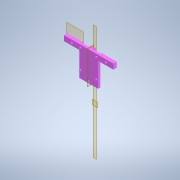
# Autodesk Inventor part: STM_Rear
Saved by Autodesk Inventor 2020 (Build 240168000, 168)
## iProperties
Created: 2022-10-27
Part Number: STM_Rear
Material: 일반
Document SubType Name: Modeling
Designer: ASUS
Density: 1 g/cm^3
Appearance: 기본값
Author: ASUS
Autodesk Inventor part; units mm, degrees
ref_plane "YZ Plane" through (0, 0, 0) normal (1, 0, 0) x (0, 1, 0)
ref_plane "작업 평면1" through (0, 0, 0) normal (0, 0, 1) x (1, 0, 0)
sketch "스케치1" plane through (0, 0, 0) normal (0, 0, 1) x (1, 0, 0)
  line L0 (18, -188.5) -> (18, 261.5) projected
  line L1 (-62, 170.2) -> (-62, 0) projected
  line L2 (-62, -188.5) -> (-62, 261.5) projected
  line L3 (163.5, 192.5) -> (-207.5, 192.5) projected
  line L4 (-32, 167.5) -> (-12, 167.5) projected
  line L5 (-12, 167.5) -> (-12, 192.5) projected
  line L6 (-32, 192.5) -> (-32, 167.5) projected
  line L7 (-12, -188.5) -> (-12, 261.5) projected
  line L8 (-32, -188.5) -> (-32, 261.5) projected
  line L9 (-32, 62) -> (-12, 62) projected
  line L10 (-62, 62.2) -> (18, 62.2)
  line L11 (18, 62.2) -> (18, 192.5)
  line L12 (18, 192.5) -> (-62, 192.5)
  line L13 (-62, 192.5) -> (-62, 62.2)
  point P0 (0, 0)
  point P1 (-62, 192.5)
  dimension "d0" = 0.2
  constraints: 8 end point, 3 point on line, 2 parallel, 1 horizontal, 1 perpendicular
  measures "d0" distance between parallel lines of L9 L10
extrude "돌출1" add sketch "스케치1" along normal blind 10 contours L10 L7 L5 L3 L0 | L10 L8 L4 L7 | L5 L4 L6 L3 | L10 L1 L2 L3 L6 L8
ref_plane "작업 평면2" through (-62, 228.54, -4.7) normal (0, 0, 1) x (0, -1, 0)
sketch "스케치2" plane through (-62, 228.54, -4.7) normal (0, 0, 1) x (0, -1, 0)
  circle A0 centre (15.0001, -54) radius 2.25 projected
  circle A1 centre (15.0001, -13) radius 2.25 projected
  line L0 (68.34, 0) -> (0, 0) projected
  line L1 (68.34, 0) -> (68.34, -67) projected
  line L2 (68.34, -67) -> (0, -67) projected
  line L3 (0, 0) -> (0, -67) projected
  circle A2 centre (15.0001, -54) radius 4 projected
  circle A3 centre (15.0001, -13) radius 4 projected
  line L4 (0, 0) -> (58.34, 0) projected
  line L5 (0, 0) -> (0, -67) projected
  line L6 (0, -67) -> (58.34, -67) projected
  line L7 (58.34, 0) -> (58.34, -67) projected
  circle A4 centre (15.0001, 134) radius 4 projected
  circle A5 centre (15.0001, 93) radius 4 projected
  line L8 (0, 80) -> (58.34, 80) projected
  line L9 (58.34, 80) -> (58.34, 147) projected
  line L10 (0, 147) -> (58.34, 147) projected
  line L11 (0, 80) -> (0, 147) projected
  line L12 (36.04, 225.5) -> (36.04, -145.5) projected
  point P0 (228.54, 62)
  point P1 (36.04, 147)
  point P2 (36.04, 80)
  point P3 (36.04, 0)
  point P4 (36.04, -67)
extrude "돌출2" add sketch "스케치2" along normal up to surface (14.7 mm away) contours L7 L2 L12 L0 | L12 L10 L9 L8
sketch "스케치3" plane through (0, 0, 10) normal (0, 0, 1) x (1, 0, 0)
  line L0 (18, 62.2) -> (18, 170.2) projected
  line L1 (85, 170.2) -> (18, 170.2) projected
  line L2 (85, 192.5) -> (85, 170.2) projected
  line L3 (-129, 192.5) -> (85, 192.5) projected
  line L4 (-129, 170.2) -> (-129, 192.5) projected
  line L5 (-62, 170.2) -> (-129, 170.2) projected
  line L6 (-62, 170.2) -> (-62, 62.2) projected
  line L7 (-62, 62.2) -> (18, 62.2) projected
  circle A0 centre (-95.5, 181.35) radius 4
  line L8 (-97.8094, 177.35) -> (-100.1188, 181.35)
  line L9 (-100.1188, 181.35) -> (-97.8094, 185.35)
  line L10 (-97.8094, 185.35) -> (-93.1906, 185.35)
  line L11 (-93.1906, 185.35) -> (-90.8812, 181.35)
  line L12 (-90.8812, 181.35) -> (-93.1906, 177.35)
  line L13 (-93.1906, 177.35) -> (-97.8094, 177.35)
  circle A1 centre (-22, 70.2) radius 4
  line L14 (-24.3094, 66.2) -> (-26.6188, 70.2)
  line L15 (-26.6188, 70.2) -> (-24.3094, 74.2)
  line L16 (-24.3094, 74.2) -> (-19.6906, 74.2)
  line L17 (-19.6906, 74.2) -> (-17.3812, 70.2)
  line L18 (-17.3812, 70.2) -> (-19.6906, 66.2)
  line L19 (-19.6906, 66.2) -> (-24.3094, 66.2)
  line L20 (18, 62.2) -> (18, 170.2) projected
  line L21 (18, 62.2) -> (-62, 62.2)
  line L22 (-62, 170.2) -> (-129, 170.2) projected
  line L23 (-129, 170.2) -> (-129, 192.5) projected
  line L24 (-62, 170.2) -> (-129, 170.2)
  line L25 (-129, 170.2) -> (-129, 192.5)
  point P0 (0, 0)
  point P1 (-95.5, 177.35)
  point P2 (-22, 66.2)
  point P3 (-129, 181.35)
  point P4 (-129, 181.35)
  point P5 (-22, 62.2)
  point P6 (-95.5, 170.2)
  dimension "d5" = 8
  dimension "d6" = 8
  dimension "d7" = 8
  constraints: 30 end point, 6 midpoint, 4 vertical alignment, 2 coincident, 2 horizontal alignment, 2 perpendicular, 1 collinear, 30 other
  measures "d7" distance from line of L7 point (-22, 70.2)
sketch "스케치4" plane through (0, 0, 0) normal (0, 0, -1) x (-1, 0, 0)
  line L0 (32, 62) -> (12, 62) projected
  line L1 (12, 62) -> (12, 198.5399) projected
  line L2 (32, 198.5399) -> (12, 198.5399) projected
  line L3 (32, 62) -> (32, 198.5399) projected
  line L4 (-18, 62.2) -> (-18, 170.2) projected
  line L5 (-85, 170.2) -> (-18, 170.2) projected
  line L6 (-85, 192.5) -> (-85, 170.2) projected
  line L7 (129, 192.5) -> (-85, 192.5) projected
  line L8 (129, 170.2) -> (129, 192.5) projected
  line L9 (62, 170.2) -> (129, 170.2) projected
  line L10 (62, 170.2) -> (62, 62.2) projected
  line L11 (62, 62.2) -> (-18, 62.2) projected
  circle A0 centre (22, 70.2) radius 2.25 projected
  point P0 (0, 0)
  point P1 (12, 62.2)
  point P2 (32, 62.2)
  point P3 (32, 192.5)
  point P4 (12, 192.5)
ref_plane "작업 평면3" through (-32, 62, -10) normal (0, 0, 1) x (1, 0, 0)
extrude "돌출4" add sketch "스케치4" along normal up to surface (10 mm away) contours L11 L1 L7 L3 | A0
ref_plane "작업 평면4" through (0, 0, 5.8) normal (0, 0, 1) x (1, 0, 0)
sketch "스케치5" plane through (0, 0, 5.8) normal (0, 0, 1) x (1, 0, 0)
  line L0 (18, 62.2) -> (18, 170.2) projected
  line L1 (85, 170.2) -> (18, 170.2) projected
  line L2 (85, 192.5) -> (85, 170.2) projected
  line L3 (-129, 192.5) -> (85, 192.5) projected
  line L4 (-129, 170.2) -> (-129, 192.5) projected
  line L5 (-62, 170.2) -> (-129, 170.2) projected
  line L6 (-62, 170.2) -> (-62, 62.2) projected
  line L7 (-62, 62.2) -> (18, 62.2) projected
  circle A0 centre (-22, 70.2) radius 4
  line L8 (-24.3094, 74.2) -> (-26.6188, 70.2) projected
  circle A1 centre (-95.5, 181.35) radius 4
  point P0 (0, 0)
  constraints: 2 centre point, 1 tangent
hole "구멍1" at (-95.5, 181.35, 5.8) direction (0, 0, -1) diameter 4.5 end through all clearance for "Socket Head Cap Screw ISO 4762" size "M4" standard "ISO"
sketch "스케치6" plane through (0, 0, 0) normal (0, 0, -1) x (-1, 0, 0)
  circle A0 centre (56.5, 98.5) radius 3
  circle A1 centre (56.5, 182.5) radius 3
  line L0 (32, 192.5) -> (62, 192.5) projected
  line L1 (62, 170.2) -> (62, 62.2) projected
  line L2 (53.0359, 98.5) -> (54.7679, 101.5)
  line L3 (54.7679, 101.5) -> (58.2321, 101.5)
  line L4 (58.2321, 101.5) -> (59.9641, 98.5)
  line L5 (59.9641, 98.5) -> (58.2321, 95.5)
  line L6 (58.2321, 95.5) -> (54.7679, 95.5)
  line L7 (54.7679, 95.5) -> (53.0359, 98.5)
  line L8 (54.7679, 179.5) -> (53.0359, 182.5)
  line L9 (53.0359, 182.5) -> (54.7679, 185.5)
  line L10 (54.7679, 185.5) -> (58.2321, 185.5)
  line L11 (58.2321, 185.5) -> (59.9641, 182.5)
  line L12 (59.9641, 182.5) -> (58.2321, 179.5)
  line L13 (58.2321, 179.5) -> (54.7679, 179.5)
  point P0 (0, 0)
  point P1 (53.9019, 97)
  point P2 (56.5, 179.5)
  point P3 (56.5, 95.5)
  dimension "d20" = 6
  dimension "d19" = 84
  dimension "d21" = 10
  dimension "d22" = 5.5
  constraints: 24 end point, 3 midpoint, 3 vertical alignment, 2 coincident, 1 horizontal, 31 other
  measures "d19" distance of point (56.5, 182.5) point (56.5, 98.5)
  measures "d21" distance from line of L0 point (56.5, 182.5)
  measures "d22" distance from line of L1 point (56.5, 98.5)
extrude "돌출5" cut sketch "스케치6" against normal blind 5.2
extrude "돌출6" cut sketch "스케치3" against normal blind 8 contours A0 | A0 L11 L12 | A0 L10 L11 | L12 L13 A0 | A0 L9 L10 | L13 L8 A0 | A0 L8 L9
sketch "스케치7" plane through (0, 0, 10) normal (0, 0, 1) x (1, 0, 0)
  line L0 (-58.2321, 101.5) -> (-59.9641, 98.5) projected
  line L1 (-59.9641, 98.5) -> (-58.2321, 95.5) projected
  line L2 (-58.2321, 95.5) -> (-54.7679, 95.5) projected
  line L3 (-54.7679, 95.5) -> (-53.0359, 98.5) projected
  line L4 (-53.0359, 98.5) -> (-54.7679, 101.5) projected
  line L5 (-54.7679, 101.5) -> (-58.2321, 101.5) projected
  line L6 (-58.2321, 185.5) -> (-59.9641, 182.5) projected
  line L7 (-59.9641, 182.5) -> (-58.2321, 179.5) projected
  line L8 (-58.2321, 179.5) -> (-54.7679, 179.5) projected
  line L9 (-54.7679, 179.5) -> (-53.0359, 182.5) projected
  line L10 (-53.0359, 182.5) -> (-54.7679, 185.5) projected
  line L11 (-54.7679, 185.5) -> (-58.2321, 185.5) projected
  line L12 (-32, 192.5) -> (-32, 62.2) projected
  line L13 (-62, 62.2) -> (-32, 62.2) projected
  line L14 (-62, 170.2) -> (-62, 62.2) projected
  line L15 (-62, 192.5) -> (-62, 170.2) projected
  line L16 (-32, 192.5) -> (-62, 192.5) projected
  point P0 (0, 0)
extrude "돌출7" add sketch "스케치7" along normal blind 5 contours L5 L4 L3 L2 L1 L0 | L11 L10 L9 L8 L7 L6
sketch "스케치8" plane through (0, 0, 15) normal (0, 0, 1) x (1, 0, 0)
  line L0 (-59.9641, 182.5) -> (-58.2321, 185.5) projected
  line L1 (-58.2321, 185.5) -> (-54.7679, 185.5) projected
  line L2 (-54.7679, 185.5) -> (-53.0359, 182.5) projected
  line L3 (-53.0359, 182.5) -> (-54.7679, 179.5) projected
  line L4 (-54.7679, 179.5) -> (-58.2321, 179.5) projected
  line L5 (-58.2321, 179.5) -> (-59.9641, 182.5) projected
  line L6 (-53.0359, 98.5) -> (-54.7679, 95.5) projected
  line L7 (-54.7679, 95.5) -> (-58.2321, 95.5) projected
  line L8 (-58.2321, 95.5) -> (-59.9641, 98.5) projected
  line L9 (-59.9641, 98.5) -> (-58.2321, 101.5) projected
  line L10 (-58.2321, 101.5) -> (-54.7679, 101.5) projected
  line L11 (-54.7679, 101.5) -> (-53.0359, 98.5) projected
  line L12 (-90.8812, 181.35) -> (-93.1906, 177.35) projected
  line L13 (-93.1906, 177.35) -> (-97.8094, 177.35) projected
  line L14 (-97.8094, 177.35) -> (-100.1188, 181.35) projected
  line L15 (-100.1188, 181.35) -> (-97.8094, 185.35) projected
  line L16 (-97.8094, 185.35) -> (-93.1906, 185.35) projected
  line L17 (-93.1906, 185.35) -> (-90.8812, 181.35) projected
  line L18 (18, 62.2) -> (18, 170.2) projected
  line L19 (85, 170.2) -> (18, 170.2) projected
  line L20 (85, 192.5) -> (85, 170.2) projected
  line L21 (-129, 192.5) -> (85, 192.5) projected
  line L22 (-129, 170.2) -> (-129, 192.5) projected
  line L23 (-62, 170.2) -> (-129, 170.2) projected
  line L24 (-62, 170.2) -> (-62, 62.2) projected
  line L25 (-62, 62.2) -> (18, 62.2) projected
  circle A0 centre (-56.5, 98.5) radius 3
  circle A1 centre (-56.5, 182.5) radius 3
  point P0 (0, 0)
  constraints: 2 centre point, 1 tangent
hole "구멍2" at (-56.5, 182.5, 15) at (-56.5, 98.5, 15) direction (0, 0, -1) diameter 3.4 end through all clearance for "Socket Head Cap Screw ISO 4762" size "M3" standard "ISO"
ref_plane "작업 평면5" through (-22, 62.2, 0) normal (-1, 0, 0) x (0, 0, 1)
mirror "미러1" about plane through (-22, 62.2, 0) normal (-1, 0, 0) of "돌출7", "구멍2", "구멍1", "돌출6", "돌출5"
sketch "스케치9" plane through (-62, 62.2, 10) normal (0, -1, 0) x (1, 0, 0)
  line L0 (0, -10) -> (30, -10) projected
  line L1 (30, -10) -> (30, -20) projected
  line L2 (50, -20) -> (30, -20) projected
  line L3 (50, -10) -> (50, -20) projected
  line L4 (50, -10) -> (80, -10) projected
  line L5 (80, -10) -> (80, 0) projected
  line L6 (0, 0) -> (80, 0) projected
  line L7 (0, -10) -> (0, 0) projected
  point P0 (62, -10)
ref_plane "작업 평면6" through (-42, 65.9601, -48) normal (0, -1, 0) x (1, 0, 0)
extrude "돌출8" cut sketch "스케치9" against normal up to surface (3.7601 mm away)
sketch "스케치12" plane through (0, 0, 10) normal (0, 0, 1) x (1, 0, 0)
  circle A0 centre (-22, 74.1601) radius 4
  line L0 (-24.3094, 70.1601) -> (-26.6188, 74.1601)
  line L1 (-26.6188, 74.1601) -> (-24.3094, 78.1601)
  line L2 (-24.3094, 78.1601) -> (-19.6906, 78.1601)
  line L3 (-19.6906, 78.1601) -> (-17.3812, 74.1601)
  line L4 (-17.3812, 74.1601) -> (-19.6906, 70.1601)
  line L5 (-19.6906, 70.1601) -> (-24.3094, 70.1601)
  point P0 (0, 0)
  point P1 (-22, 70.1601)
  constraints: 12 end point, 1 coincident, 1 midpoint, 1 vertical alignment, 16 other
extrude "돌출9" cut sketch "스케치12" against normal blind 5
sketch "스케치13" plane through (0, 0, 5) normal (0, 0, 1) x (1, 0, 0)
  line L0 (-26.6188, 74.1601) -> (-24.3094, 78.1601) projected
  line L1 (-24.3094, 78.1601) -> (-19.6906, 78.1601) projected
  line L2 (-19.6906, 78.1601) -> (-17.3812, 74.1601) projected
  line L3 (-17.3812, 74.1601) -> (-19.6906, 70.1601) projected
  line L4 (-19.6906, 70.1601) -> (-24.3094, 70.1601) projected
  line L5 (-24.3094, 70.1601) -> (-26.6188, 74.1601) projected
  line L6 (-62, 65.9601) -> (18, 65.9601) projected
  line L7 (18, 65.9601) -> (18, 170.2) projected
  line L8 (85, 170.2) -> (18, 170.2) projected
  line L9 (85, 192.5) -> (85, 170.2) projected
  line L10 (-129, 192.5) -> (85, 192.5) projected
  line L11 (-129, 170.2) -> (-129, 192.5) projected
  line L12 (-62, 170.2) -> (-129, 170.2) projected
  line L13 (-62, 170.2) -> (-62, 65.9601) projected
  line L14 (9.0359, 182.5) -> (10.7679, 185.5) projected
  line L15 (10.7679, 185.5) -> (14.2321, 185.5) projected
  line L16 (14.2321, 185.5) -> (15.9641, 182.5) projected
  line L17 (15.9641, 182.5) -> (14.2321, 179.5) projected
  line L18 (14.2321, 179.5) -> (10.7679, 179.5) projected
  line L19 (10.7679, 179.5) -> (9.0359, 182.5) projected
  line L20 (10.7679, 101.5) -> (14.2321, 101.5) projected
  line L21 (14.2321, 101.5) -> (15.9641, 98.5) projected
  line L22 (15.9641, 98.5) -> (14.2321, 95.5) projected
  line L23 (14.2321, 95.5) -> (10.7679, 95.5) projected
  line L24 (10.7679, 95.5) -> (9.0359, 98.5) projected
  line L25 (9.0359, 98.5) -> (10.7679, 101.5) projected
  line L26 (49.1906, 177.35) -> (46.8812, 181.35) projected
  line L27 (46.8812, 181.35) -> (49.1906, 185.35) projected
  line L28 (49.1906, 185.35) -> (53.8094, 185.35) projected
  line L29 (53.8094, 185.35) -> (56.1188, 181.35) projected
  line L30 (56.1188, 181.35) -> (53.8094, 177.35) projected
  line L31 (53.8094, 177.35) -> (49.1906, 177.35) projected
  line L32 (-54.7679, 185.5) -> (-53.0359, 182.5) projected
  line L33 (-53.0359, 182.5) -> (-54.7679, 179.5) projected
  line L34 (-54.7679, 179.5) -> (-58.2321, 179.5) projected
  line L35 (-58.2321, 179.5) -> (-59.9641, 182.5) projected
  line L36 (-59.9641, 182.5) -> (-58.2321, 185.5) projected
  line L37 (-58.2321, 185.5) -> (-54.7679, 185.5) projected
  line L38 (-58.2321, 101.5) -> (-54.7679, 101.5) projected
  line L39 (-54.7679, 101.5) -> (-53.0359, 98.5) projected
  line L40 (-53.0359, 98.5) -> (-54.7679, 95.5) projected
  line L41 (-54.7679, 95.5) -> (-58.2321, 95.5) projected
  line L42 (-58.2321, 95.5) -> (-59.9641, 98.5) projected
  line L43 (-59.9641, 98.5) -> (-58.2321, 101.5) projected
  line L44 (-90.8812, 181.35) -> (-93.1906, 177.35) projected
  line L45 (-93.1906, 177.35) -> (-97.8094, 177.35) projected
  line L46 (-97.8094, 177.35) -> (-100.1188, 181.35) projected
  line L47 (-100.1188, 181.35) -> (-97.8094, 185.35) projected
  line L48 (-97.8094, 185.35) -> (-93.1906, 185.35) projected
  line L49 (-93.1906, 185.35) -> (-90.8812, 181.35) projected
  circle A0 centre (-22, 74.1601) radius 2.25
  point P0 (0, 0)
  constraints: 1 centre point, 2 other
hole "구멍3" at (-22, 74.1601, 5) direction (0, 0, -1) diameter 4.5 end through all
sketch "스케치14" plane through (85, 170.2, -4.7) normal (1, 0, 0) x (0, 0, -1)
  line L0 (-14.7, 22.3) -> (-14.7, 0) projected
  line L1 (0, 0) -> (-14.7, 0) projected
  line L2 (0, 0) -> (0, 22.3) projected
  line L3 (0, 22.3) -> (-14.7, 22.3) projected
  point P0 (-4.7, -170.2)
extrude "돌출10" cut sketch "스케치14" against normal blind 1
sketch "스케치16" plane through (-129, 170.2, -4.7) normal (-1, 0, 0) x (0, 0, 1)
  line L0 (14.7, 0) -> (14.7, 22.3) projected
  line L1 (0, 22.3) -> (14.7, 22.3) projected
  line L2 (0, 22.3) -> (0, 0) projected
  line L3 (0, 0) -> (14.7, 0) projected
  point P0 (4.7, -170.2)
extrude "돌출11" cut sketch "스케치16" against normal blind 1
equation "\"d25\" = d6"
